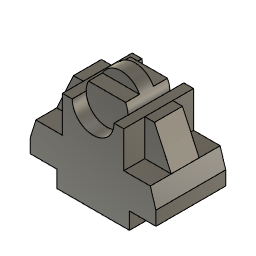
Sketch8_Final v1 (Autodesk Fusion 360 design; units mm, degrees)
Autodesk Fusion 360 part; units mm, degrees
sketch "Sketch1" plane through (0, 0, 0) normal (0, 1, 0) x (1, 0, 0)
  line L0 (0, 0) -> (26, 0)
  line L1 (26, 0) -> (26, -12)
  line L2 (26, -12) -> (45, -12)
  line L3 (45, -12) -> (45, -22)
  line L4 (22, -35) -> (41, -35)
  line L5 (41, -35) -> (45, -22)
  line L6 (0, 0) -> (0, -85)
  line L7 (22, -35) -> (22, -61)
  line L8 (22, -61) -> (15, -61)
  arc A0 (15, -61) -> (0, -46) centre (0, -61) ccw
  arc A1 (0, -46) -> (-15, -61) centre (0, -61) ccw
  line L9 (-22, -61) -> (-15, -61)
  line L10 (-22, -35) -> (-22, -61)
  line L11 (-22, -35) -> (-41, -35)
  line L12 (-41, -35) -> (-45, -22)
  line L13 (-45, -12) -> (-45, -22)
  line L14 (-26, -12) -> (-45, -12)
  line L15 (-26, 0) -> (-26, -12)
  line L16 (0, 0) -> (-26, 0)
  dimension "d1" = 26
  dimension "d2" = 12
  dimension "d3" = 19
  dimension "d4" = 10
  dimension "d9" = 19
  dimension "d30" = 26
  dimension "d31" = 7
  dimension "d32" = 30
  constraint coincident L0.start L6.start
  constraint perpendicular L0 L6
  constraint perpendicular L7 L8
  constraint coincident L6 A0.centre
  constraint coincident L6 A0.end
  constraint symmetric L0.start L6 L16.start
  constraint symmetric L0.end L6 L15.start
  constraint symmetric L1.end L6 L14.start
  constraint symmetric L2.end L6 L13.start
  constraint symmetric L3.end L6 L12.end
  constraint symmetric L4.start L6 L10.start
  constraint symmetric L4.end L6 L11.end
  constraint symmetric L6 L7.end L9.start
  constraint symmetric L6 L8.end A1.end
  constraint symmetric L6 A0 A1
  constraint symmetric L6 A0.end A1.start
  measures "d1" distance of L0.start L0.end
  measures "d2" distance of L0.end L1.end
  measures "d3" distance of L1.end L2.end
  measures "d4" distance of L2.end L3.end
  measures "d9" distance of L4.start L4.end
  measures "d30" distance of L4.start L7.end
  measures "d31" distance of L7.end L8.end
  measures "d32" diameter of A0
sketch "Sketch2" plane through (0, 0, 0) normal (0, 1, 0) x (1, 0, 0)
  line L0 (-22, -35) -> (-22.036091, -60.999975)
  line L1 (-22, -35) -> (-40.999999, -34.995353)
  line L2 (-22.036091, -60.999975) -> (-29.036084, -60.990258)
  line L3 (-29.036084, -60.990258) -> (-40.999999, -34.995353)
  line L4 (0, 0) -> (-0.019544, -79.90912)
  line L5 (22.00625, -61.010747) -> (29.006247, -61.004454)
  line L6 (29.006247, -61.004454) -> (40.982876, -35.015404)
  line L7 (21.982877, -35.010757) -> (40.982876, -35.015404)
  line L8 (21.982877, -35.010757) -> (22.00625, -61.010747)
  dimension "d19" = 19
  dimension "d22" = 26
  dimension "d27" = 7
  constraint perpendicular L0 L2
  constraint coincident L4.start origin
  constraint perpendicular L1 L4
sketch "Sketch4" plane through (0, 0, 0) normal (0, 1, 0) x (1, 0, 0)
  circle A0 centre (0, -61.000001) radius 15
  dimension "d33" = 30
  measures "d33" diameter of A0
extrude "Extrude4" add sketch "Sketch1" along normal mid plane 50 contours L0 L1 L2 L3 L4 L5 L6 L7 L8 A0 | L6 A1 L9 L10 L11 L12 L13 L14 L15 L16 picked at (7.333333, -27) picked at (-7.333333, -27)
extrude "Extrude5" add sketch "Sketch2" along normal mid plane 20 contours L0 L1 L2 L3 | L5 L6 L7 L8 picked at (-30.678695, -43.66187) picked at (30.657333, -43.676872)
extrude "Extrude6" add sketch "Sketch4" along normal mid plane 30 contours A0 picked at (-6.730054, -63.16942)
sketch "Sketch5" plane through (0, 0, 0) normal (1, 0, 0) x (0, 1, 0)
  line L0 (0, 0) -> (0, 76.000001)
  line L1 (15, 76.000001) -> (5, 76.000001)
  line L2 (5, 76.000001) -> (5, 68.000001)
  line L3 (5, 68.000001) -> (15, 68.000001)
  line L4 (15, 68.000001) -> (15, 76.000001)
  line L5 (-15, 76.000001) -> (-5, 76.000001)
  line L6 (-5, 76.000001) -> (-5, 68.000001)
  line L7 (-5, 68.000001) -> (-15, 68.000001)
  line L8 (-15, 68.000001) -> (-15, 76.000001)
  dimension "d43" = 76
  dimension "d44" = 10
  constraint coincident L0.start origin
  constraint vertical L0
  constraint horizontal L1
  constraint vertical L2
  constraint horizontal L3
  constraint vertical L4
extrude "Extrude7" cut sketch "Sketch5" along normal mid plane 44 contours L1 L2 L3 L4 | L5 L6 L7 L8 picked at (8.333333, 73.333334) picked at (-11.666667, 73.333334)
extrude "Extrude1" [rolled back] along distance 25 taper angle 0
extrude "Extrude2" [rolled back] along distance 10 taper angle 0
extrude "Extrude3" [rolled back] along distance 10 taper angle 0
